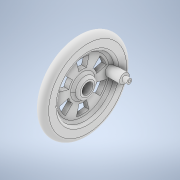
# Autodesk Inventor part: Vasiletrainwheel
Saved by Autodesk Inventor 2020 (Build 240168000, 168)
## iProperties
Created: 2020-04-30
Part Number: Vasiletrainwheel
Material: ABS Plastic
Document SubType Name: Modeling
Designer: al
Density: 1.06 g/cm^3
Appearance: Smooth - White
Author: al
Autodesk Inventor part; units mm, degrees
ref_plane "YZ Plane" through (0, 0, 0) normal (1, 0, 0) x (0, 1, 0)
ref_plane "XZ Plane" through (0, 0, 0) normal (0, 1, 0) x (-1, 0, 0)
ref_plane "XY Plane" through (0, 0, 0) normal (0, 0, 1) x (1, 0, 0)
sketch "Sketch1" plane through (0, 0, 0) normal (0, 0, 1) x (1, 0, 0)
  line L0 (-11.8178, 6.8348) -> (-5.4678, 6.8348)
  line L1 (-5.4678, 6.8348) -> (-5.4678, 10.0098)
  line L2 (-5.4678, 10.0098) -> (7.2322, 10.0098)
  line L3 (7.2322, 10.0098) -> (7.2322, 6.8348)
  line L4 (7.2322, 6.8348) -> (10.0262, 6.8348)
  line L5 (10.0262, 6.8348) -> (10.0262, 13.1848)
  line L6 (10.0262, 13.1848) -> (-11.8178, 13.1848)
  line L7 (13.5822, 11.2511) -> (13.5822, 4.7509)
  arc A0 (-11.8178, 13.1848) -> (-11.8178, 6.8348) centre (-11.8178, 10.0098) ccw
  point P0 (0, 0)
  dimension "d0" = 3.556
  dimension "d1" = 6.35
  dimension "d2" = 19.05
  dimension "d4" = 6.35
  dimension "d5" = 3.175
  dimension "d6" = 6.35
  constraints: 16 end point, 5 perpendicular, 3 point on line, 2 point on circle, 1 centre point, 1 vertical
  measures "d0" distance between parallel lines of L5 L7
  measures "d1" distance between parallel lines of L7 L3
  measures "d2" distance between parallel lines of L7 L1
  measures "d4" distance from line of L6 L0.start
  measures "d5" distance between parallel lines of L6 L2
  measures "d6" diameter of A0
revolve "Revolution1" add sketch "Sketch1" angle 360 about axis through (13.5822, 11.2511, 0) along (0, -1, 0)
fillet "Fillet1" radius 1.6002 4 edges at (19.9322, 6.8348, 0) (19.9322, 10.0098, 0) (32.6322, 10.0098, 0) (32.6322, 6.8348, 0)
sketch "Sketch2" plane through (13.5822, 10.0098, 0) normal (0, -1, 0) x (1, 0, 0)
  circle A0 centre (17.78, 0) radius 3.175
  circle A1 centre (17.78, 0) radius 1.5875
  circle A2 centre (0, 0) radius 4.7498 projected
  point P0 (-13.5822, 0)
  dimension "d9" = 6.35
  dimension "d10" = 3.175
  dimension "d11" = 17.78
  constraints: 2 centre point, 1 coincident, 1 other
  measures "d9" diameter of A0
  measures "d10" diameter of A1
  measures "d11" distance of A2.centre A0.centre
extrude "Extrusion1" add sketch "Sketch2" along normal blind 9.525 contours A0 | A1
extrude "Extrusion2" add sketch "Sketch2" along normal blind 12.7 contours A1
sketch "Sketch3" plane through (31.3622, -2.6902, 0) normal (0, -1, 0) x (1, 0, 0)
  circle A0 centre (0, 0) radius 0.7937
  point P0 (-31.3622, 0)
  dimension "d16" = 1.5875
  constraints: 1 centre point
  measures "d16" diameter of A0
extrude "Extrusion3" cut sketch "Sketch3" against normal blind 6.35
sketch "Sketch4" plane through (13.5822, 10.0098, 0) normal (0, -1, 0) x (1, 0, 0)
  circle A0 centre (0, 0) radius 9.398
  circle A1 centre (0, 0) radius 16.002
  line L0 (0, 0) -> (0, 17.4498)
  arc A2 (17.1694, 3.1157) -> (17.1694, -3.1157) centre (0, 0) ccw projected
  line L1 (-2.4324, 9.0778) -> (-4.1416, 15.4567)
  line L2 (2.4324, 9.0778) -> (4.1416, 15.4567)
  point P0 (-13.5822, 0)
  dimension "d19" = 18.796
  dimension "d20" = 32.004
  dimension "d21" = 15
  dimension "d22" = 15
  constraints: 6 end point, 5 point on circle, 2 centre point, 1 coincident, 1 vertical
  measures "d19" diameter of A0
  measures "d20" diameter of A1
  measures "d21" angle of L1 L0
  measures "d22" angle of L0 L2
extrude "Extrusion4" cut sketch "Sketch4" against normal blind 6.35 contours A0 L0 A1 L2 | L1 A1 L0 A0
pattern_circular "Circular Pattern1" count 6 over 360 about axis through (13.5822, 10.0098, 0) along (0, 1, 0) of "Extrusion4"
body "Solid1"
